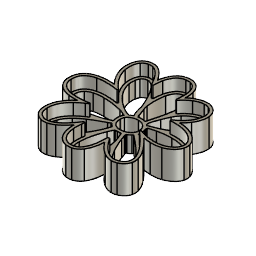
Flower v6 (Autodesk Fusion 360 design; units mm, degrees)
Autodesk Fusion 360 part; units mm, degrees
(part 1 of 2)
sketch "Sketch1" plane through (0, 0, 0) normal (0, 0, 1) x (1, 0, 0)
  spline S0 degree 3 poles (24.398238, -49.491999) (21.853797, -49.043086) (20.145962, -46.595318) (19.808691, -42.913987) knots 0 0 0 0 1 1 1 1
  spline S1 degree 3 poles (19.808691, -42.913987) (19.738303, -42.145705) (19.777142, -40.404034) (19.883263, -39.569933) knots 0 0 0 0 1 1 1 1
  spline S2 degree 3 poles (19.883263, -39.569933) (19.974868, -38.849932) (20.169101, -37.728624) (20.298509, -37.172733) knots 0 0 0 0 1 1 1 1
  spline S3 degree 3 poles (20.298509, -37.172733) (20.350138, -36.950954) (20.383684, -36.760803) (20.373056, -36.750176) knots 0 0 0 0 1 1 1 1
  spline S4 degree 3 poles (20.373056, -36.750176) (20.362429, -36.739548) (20.207496, -36.975057) (20.02876, -37.273529) knots 0 0 0 0 1 1 1 1
  spline S5 degree 3 poles (20.02876, -37.273529) (18.11849, -40.463515) (15.8391, -43.11864) (13.903666, -44.40829) knots 0 0 0 0 1 1 1 1
  spline S6 degree 3 poles (13.903666, -44.40829) (13.13197, -44.9225) (12.4509, -45.23528) (11.669465, -45.434349) knots 0 0 0 0 1 1 1 1
  spline S7 degree 3 poles (11.669465, -45.434349) (11.12034, -45.574233) (10.211189, -45.587693) (9.705467, -45.463417) knots 0 0 0 0 1 1 1 1
  spline S8 degree 3 poles (9.705467, -45.463417) (8.958562, -45.27987) (8.179688, -44.834118) (7.596024, -44.256169) knots 0 0 0 0 1 1 1 1
  spline S9 degree 3 poles (7.596024, -44.256169) (6.902032, -43.568975) (6.551135, -42.561718) (6.474, -41.035376) knots 0 0 0 0 1 1 1 1
  spline S10 degree 3 poles (6.474, -41.035376) (6.338825, -38.360532) (7.582333, -35.682392) (10.063361, -33.304973) knots 0 0 0 0 1 1 1 1
  spline S11 degree 3 poles (10.063361, -33.304973) (10.912309, -32.49148) (11.717344, -31.841911) (12.942719, -30.981678) knots 0 0 0 0 1 1 1 1
  spline S12 degree 3 poles (12.942719, -30.981678) (13.486476, -30.599953) (14.664879, -29.844231) (14.781144, -29.80268) knots 0 0 0 0 1 1 1 1
  spline S13 degree 3 poles (14.781144, -29.80268) (14.813838, -29.790993) (14.829778, -29.770067) (14.816565, -29.756169) knots 0 0 0 0 1 1 1 1
  spline S14 degree 3 poles (14.816565, -29.756169) (14.803352, -29.742275) (14.554706, -29.781213) (14.264021, -29.842704) knots 0 0 0 0 1 1 1 1
  spline S15 degree 3 poles (14.264021, -29.842704) (13.428167, -30.019514) (12.387035, -30.189924) (11.439225, -30.305062) knots 0 0 0 0 1 1 1 1
  spline S16 degree 3 poles (11.439225, -30.305062) (10.694335, -30.39555) (10.318137, -30.411456) (8.906743, -30.412145) knots 0 0 0 0 1 1 1 1
  spline S17 degree 3 poles (8.906743, -30.412145) (7.429716, -30.412867) (7.176998, -30.401447) (6.587244, -30.307359) knots 0 0 0 0 1 1 1 1
  spline S18 degree 3 poles (6.587244, -30.307359) (4.61966, -29.993447) (3.257425, -29.398503) (2.302777, -28.436158) knots 0 0 0 0 1 1 1 1
  spline S19 degree 3 poles (2.302777, -28.436158) (1.404569, -27.53071) (0.964594, -26.480042) (0.898892, -25.083663) knots 0 0 0 0 1 1 1 1
  spline S20 degree 3 poles (0.898892, -25.083663) (0.752423, -21.97074) (2.495588, -19.901678) (5.951833, -19.086041) knots 0 0 0 0 1 1 1 1
  spline S21 degree 3 poles (5.951833, -19.086041) (8.285184, -18.535394) (11.801198, -18.57942) (15.197135, -19.201807) knots 0 0 0 0 1 1 1 1
  spline S22 degree 3 poles (15.197135, -19.201807) (15.472515, -19.252277) (15.706188, -19.285206) (15.71641, -19.274984) knots 0 0 0 0 1 1 1 1
  spline S23 degree 3 poles (15.71641, -19.274984) (15.726633, -19.264761) (15.663483, -19.206281) (15.576077, -19.145026) knots 0 0 0 0 1 1 1 1
  spline S24 degree 3 poles (15.576077, -19.145026) (15.173173, -18.862672) (14.403009, -18.229035) (13.855618, -17.729554) knots 0 0 0 0 1 1 1 1
  spline S25 degree 3 poles (13.855618, -17.729554) (11.319411, -15.415325) (9.535422, -12.521165) (8.985416, -9.828637) knots 0 0 0 0 1 1 1 1
  spline S26 degree 3 poles (8.985416, -9.828637) (8.541535, -7.655641) (8.849932, -5.515577) (9.799961, -4.176243) knots 0 0 0 0 1 1 1 1
  spline S27 degree 3 poles (9.799961, -4.176243) (10.248531, -3.543857) (11.043643, -3.01215) (11.885678, -2.781482) knots 0 0 0 0 1 1 1 1
  spline S28 degree 3 poles (11.885678, -2.781482) (12.362987, -2.650728) (13.37267, -2.662599) (13.879642, -2.804928) knots 0 0 0 0 1 1 1 1
  spline S29 degree 3 poles (13.879642, -2.804928) (16.035873, -3.410271) (18.317612, -5.96279) (20.405058, -10.10473) knots 0 0 0 0 1 1 1 1
  spline S30 degree 3 poles (20.405058, -10.10473) (20.621428, -10.534053) (20.809268, -10.885434) (20.822481, -10.885577) knots 0 0 0 0 1 1 1 1
  spline S31 degree 3 poles (20.822481, -10.885577) (20.835694, -10.88572) (20.839472, -10.577696) (20.830878, -10.201083) knots 0 0 0 0 1 1 1 1
  spline S32 degree 3 poles (20.830878, -10.201083) (20.800341, -8.862913) (20.965717, -7.099114) (21.2307, -5.936803) knots 0 0 0 0 1 1 1 1
  spline S33 degree 3 poles (21.2307, -5.936803) (21.953131, -2.767962) (23.46365, -0.994904) (25.819403, -0.550548) knots 0 0 0 0 1 1 1 1
  spline S34 degree 3 poles (25.819403, -0.550548) (26.276354, -0.464355) (27.303759, -0.478399) (27.762296, -0.577105) knots 0 0 0 0 1 1 1 1
  spline S35 degree 3 poles (27.762296, -0.577105) (29.380756, -0.925504) (30.471677, -2.110585) (30.979854, -4.072385) knots 0 0 0 0 1 1 1 1
  spline S36 degree 3 poles (30.979854, -4.072385) (31.228572, -5.032546) (31.272789, -5.499233) (31.272596, -7.162009) knots 0 0 0 0 1 1 1 1
  spline S37 degree 3 poles (31.272596, -7.162009) (31.272402, -8.704189) (31.219619, -9.467197) (31.030104, -10.666355) knots 0 0 0 0 1 1 1 1
  spline S38 degree 3 poles (31.030104, -10.666355) (30.971872, -11.03482) (30.969098, -11.198786) (31.022394, -11.12191) knots 0 0 0 0 1 1 1 1
  spline S39 degree 3 poles (31.022394, -11.12191) (31.030028, -11.1109) (31.140908, -10.92892) (31.268795, -10.717512) knots 0 0 0 0 1 1 1 1
  spline S40 degree 3 poles (31.268795, -10.717512) (32.09923, -9.344737) (33.682992, -7.788682) (35.140585, -6.913456) knots 0 0 0 0 1 1 1 1
  spline S41 degree 3 poles (35.140585, -6.913456) (36.521936, -6.084012) (37.649445, -5.70804) (38.888276, -5.663775) knots 0 0 0 0 1 1 1 1
  spline S42 degree 3 poles (38.888276, -5.663775) (39.709456, -5.634433) (40.245182, -5.722796) (40.924003, -5.999548) knots 0 0 0 0 1 1 1 1
  spline S43 degree 3 poles (40.924003, -5.999548) (42.412514, -6.606408) (43.266225, -7.780936) (43.456796, -9.48414) knots 0 0 0 0 1 1 1 1
  spline S44 degree 3 poles (43.456796, -9.48414) (43.616225, -10.909023) (42.996088, -13.033743) (41.979428, -14.545917) knots 0 0 0 0 1 1 1 1
  spline S45 degree 3 poles (41.979428, -14.545917) (41.293675, -15.565904) (40.264162, -16.673275) (39.248628, -17.483241) knots 0 0 0 0 1 1 1 1
  spline S46 degree 3 poles (39.248628, -17.483241) (38.697195, -17.92305) (37.559702, -18.70613) (37.002416, -19.02959) knots 0 0 0 0 1 1 1 1
  spline S47 degree 3 poles (37.002416, -19.02959) (36.824039, -19.133123) (36.678096, -19.236237) (36.678096, -19.258731) knots 0 0 0 0 1 1 1 1
  spline S48 degree 3 poles (36.678096, -19.258731) (36.678096, -19.281227) (36.695612, -19.288805) (36.717023, -19.275573) knots 0 0 0 0 1 1 1 1
  spline S49 degree 3 poles (36.717023, -19.275573) (36.738434, -19.262341) (37.173133, -19.217823) (37.68302, -19.176643) knots 0 0 0 0 1 1 1 1
  spline S50 degree 3 poles (37.68302, -19.176643) (42.00013, -18.827983) (45.508277, -19.629245) (47.812293, -21.490171) knots 0 0 0 0 1 1 1 1
  spline S51 degree 3 poles (47.812293, -21.490171) (48.837616, -22.318308) (49.53917, -23.300587) (49.803184, -24.277686) knots 0 0 0 0 1 1 1 1
  spline S52 degree 3 poles (49.803184, -24.277686) (49.942622, -24.793725) (49.943332, -25.611328) (49.80482, -26.123575) knots 0 0 0 0 1 1 1 1
  spline S53 degree 3 poles (49.80482, -26.123575) (49.3646, -27.751308) (47.772047, -29.18037) (45.585744, -29.909516) knots 0 0 0 0 1 1 1 1
  spline S54 degree 3 poles (45.585744, -29.909516) (44.371551, -30.314458) (43.211242, -30.465773) (41.609147, -30.428102) knots 0 0 0 0 1 1 1 1
  spline S55 degree 3 poles (41.609147, -30.428102) (40.042242, -30.391257) (38.585558, -30.162583) (36.798241, -29.672875) knots 0 0 0 0 1 1 1 1
  spline S56 degree 3 poles (36.798241, -29.672875) (36.104288, -29.482739) (34.502045, -28.970831) (34.011496, -28.782527) knots 0 0 0 0 1 1 1 1
  spline S57 degree 3 poles (34.011496, -28.782527) (33.926302, -28.749826) (33.923577, -28.753712) (33.987472, -28.816798) knots 0 0 0 0 1 1 1 1
  spline S58 degree 3 poles (33.987472, -28.816798) (34.027112, -28.855936) (34.286566, -29.080518) (34.56404, -29.315872) knots 0 0 0 0 1 1 1 1
  spline S59 degree 3 poles (34.56404, -29.315872) (37.459824, -31.772092) (40.176255, -34.522567) (41.680793, -36.521819) knots 0 0 0 0 1 1 1 1
  spline S60 degree 3 poles (41.680793, -36.521819) (42.91714, -38.164698) (43.5687, -39.364673) (43.935882, -40.675021) knots 0 0 0 0 1 1 1 1
  spline S61 degree 3 poles (43.935882, -40.675021) (44.082376, -41.197812) (44.118476, -42.215448) (44.008123, -42.711464) knots 0 0 0 0 1 1 1 1
  spline S62 degree 3 poles (44.008123, -42.711464) (43.761857, -43.818382) (42.875081, -44.768754) (41.595179, -45.297459) knots 0 0 0 0 1 1 1 1
  spline S63 degree 3 poles (41.595179, -45.297459) (41.00791, -45.540045) (40.577769, -45.62411) (39.930185, -45.622861) knots 0 0 0 0 1 1 1 1
  spline S64 degree 3 poles (39.930185, -45.622861) (38.88069, -45.620843) (37.959139, -45.323304) (36.774015, -44.603896) knots 0 0 0 0 1 1 1 1
  spline S65 degree 3 poles (36.774015, -44.603896) (34.502488, -43.225002) (32.467553, -40.903967) (30.578279, -37.537086) knots 0 0 0 0 1 1 1 1
  spline S66 degree 3 poles (30.578279, -37.537086) (30.492135, -37.383568) (30.414524, -37.265095) (30.405808, -37.273811) knots 0 0 0 0 1 1 1 1
  spline S67 degree 3 poles (30.405808, -37.273811) (30.397093, -37.282526) (30.409562, -37.559482) (30.433518, -37.889264) knots 0 0 0 0 1 1 1 1
  spline S68 degree 3 poles (30.433518, -37.889264) (30.457475, -38.219047) (30.477736, -39.033089) (30.478545, -39.698245) knots 0 0 0 0 1 1 1 1
  spline S69 degree 3 poles (30.478545, -39.698245) (30.482926, -43.298639) (29.92491, -45.894977) (28.777152, -47.61447) knots 0 0 0 0 1 1 1 1
  spline S70 degree 3 poles (28.777152, -47.61447) (28.158581, -48.54117) (27.313864, -49.174865) (26.365085, -49.423963) knots 0 0 0 0 1 1 1 1
  spline S71 degree 3 poles (26.365085, -49.423963) (25.870005, -49.553947) (24.933082, -49.586358) (24.398238, -49.491999) knots 0 0 0 0 1 1 1 1
  spline S72 degree 3 poles (25.893389, -48.240956) (26.856708, -47.993406) (27.578922, -47.344708) (28.138373, -46.224488) knots 0 0 0 0 1 1 1 1
  spline S73 degree 3 poles (28.138373, -46.224488) (29.483804, -43.53045) (29.645761, -38.006142) (28.50532, -33.708159) knots 0 0 0 0 1 1 1 1
  spline S74 degree 3 poles (28.50532, -33.708159) (28.272808, -32.831887) (28.203024, -32.626149) (27.861593, -31.810289) knots 0 0 0 0 1 1 1 1
  spline S75 degree 3 poles (27.861593, -31.810289) (27.684648, -31.387473) (27.399443, -30.695591) (27.227805, -30.272775) knots 0 0 0 0 1 1 1 1
  spline S76 degree 3 poles (27.227805, -30.272775) (27.056167, -29.849959) (26.901488, -29.489847) (26.884078, -29.47253) knots 0 0 0 0 1 1 1 1
  spline S77 degree 3 poles (26.884078, -29.47253) (26.866667, -29.455214) (26.711883, -29.473809) (26.540113, -29.513859) knots 0 0 0 0 1 1 1 1
  spline S78 degree 3 poles (26.540113, -29.513859) (26.333701, -29.561986) (25.922313, -29.59076) (25.326842, -29.598728) knots 0 0 0 0 1 1 1 1
  line L0 (25.326842, -29.598728) -> (24.425878, -29.610781)
  line L1 (24.425878, -29.610781) -> (24.22792, -29.835671)
  spline S79 degree 3 poles (24.22792, -29.835671) (24.011927, -30.081055) (23.804667, -30.524475) (23.248818, -31.930408) knots 0 0 0 0 1 1 1 1
  spline S80 degree 3 poles (23.248818, -31.930408) (21.722692, -35.790505) (21.010933, -38.900581) (21.011151, -41.708039) knots 0 0 0 0 1 1 1 1
  spline S81 degree 3 poles (21.011151, -41.708039) (21.011248, -43.081883) (21.14664, -44.015287) (21.501171, -45.086507) knots 0 0 0 0 1 1 1 1
  spline S82 degree 3 poles (21.501171, -45.086507) (21.677795, -45.620178) (22.090949, -46.450466) (22.350903, -46.794158) knots 0 0 0 0 1 1 1 1
  spline S83 degree 3 poles (22.350903, -46.794158) (22.951009, -47.587572) (23.718529, -48.09455) (24.573472, -48.262253) knots 0 0 0 0 1 1 1 1
  spline S84 degree 3 poles (24.573472, -48.262253) (24.922627, -48.330746) (25.585621, -48.320048) (25.893389, -48.240956) knots 0 0 0 0 1 1 1 1
  spline S85 degree 3 poles (40.858217, -44.247785) (42.279715, -43.779561) (43.001971, -42.786936) (42.834794, -41.531295) knots 0 0 0 0 1 1 1 1
  spline S86 degree 3 poles (42.834794, -41.531295) (42.633431, -40.018898) (41.504457, -38.100328) (39.382049, -35.663735) knots 0 0 0 0 1 1 1 1
  spline S87 degree 3 poles (39.382049, -35.663735) (38.669928, -34.846195) (36.349413, -32.536002) (35.284727, -31.584633) knots 0 0 0 0 1 1 1 1
  spline S88 degree 3 poles (35.284727, -31.584633) (33.749397, -30.212716) (32.214967, -28.941282) (30.775134, -27.847968) knots 0 0 0 0 1 1 1 1
  line L2 (30.775134, -27.847968) -> (30.181399, -27.397126)
  line L3 (30.181399, -27.397126) -> (29.838211, -27.764149)
  spline S89 degree 3 poles (29.838211, -27.764149) (29.469278, -28.158707) (29.03465, -28.501906) (28.578775, -28.75865) knots 0 0 0 0 1 1 1 1
  spline S90 degree 3 poles (28.578775, -28.75865) (28.422061, -28.846909) (28.286356, -28.924875) (28.27721, -28.931907) knots 0 0 0 0 1 1 1 1
  spline S91 degree 3 poles (28.27721, -28.931907) (28.268063, -28.938939) (28.402431, -29.340808) (28.575805, -29.824947) knots 0 0 0 0 1 1 1 1
  spline S92 degree 3 poles (28.575805, -29.824947) (28.749179, -30.309086) (29.007392, -31.061951) (29.149616, -31.497982) knots 0 0 0 0 1 1 1 1
  spline S93 degree 3 poles (29.149616, -31.497982) (29.589068, -32.845269) (30.956889, -35.77027) (31.924461, -37.431827) knots 0 0 0 0 1 1 1 1
  spline S94 degree 3 poles (31.924461, -37.431827) (33.535773, -40.198841) (35.232289, -42.134083) (37.111751, -43.34905) knots 0 0 0 0 1 1 1 1
  spline S95 degree 3 poles (37.111751, -43.34905) (38.635016, -44.333756) (39.77036, -44.60611) (40.858217, -44.247785) knots 0 0 0 0 1 1 1 1
  spline S96 degree 3 poles (11.005336, -44.276327) (12.706116, -44.048754) (14.648516, -42.571407) (16.719465, -39.930288) knots 0 0 0 0 1 1 1 1
  spline S97 degree 3 poles (16.719465, -39.930288) (18.856844, -37.204452) (20.936605, -33.436523) (21.983766, -30.392893) knots 0 0 0 0 1 1 1 1
  spline S98 degree 3 poles (21.983766, -30.392893) (22.150992, -29.906842) (22.408043, -29.005374) (22.408043, -28.904968) knots 0 0 0 0 1 1 1 1
  spline S99 degree 3 poles (22.408043, -28.904968) (22.408043, -28.885176) (22.287608, -28.78902) (22.140408, -28.691283) knots 0 0 0 0 1 1 1 1
  spline S100 degree 3 poles (22.140408, -28.691283) (21.993209, -28.593549) (21.695916, -28.334201) (21.479758, -28.114959) knots 0 0 0 0 1 1 1 1
  line L4 (21.479758, -28.114959) -> (21.086741, -27.716331)
  line L5 (21.086741, -27.716331) -> (20.846504, -27.859244)
  spline S101 degree 3 poles (20.846504, -27.859244) (20.714374, -27.937846) (20.292759, -28.164898) (19.909582, -28.363802) knots 0 0 0 0 1 1 1 1
  spline S102 degree 3 poles (19.909582, -28.363802) (17.754742, -29.482369) (15.357081, -30.859413) (14.095855, -31.70279) knots 0 0 0 0 1 1 1 1
  spline S103 degree 3 poles (14.095855, -31.70279) (12.638315, -32.677443) (11.799362, -33.354871) (10.753846, -34.401361) knots 0 0 0 0 1 1 1 1
  spline S104 degree 3 poles (10.753846, -34.401361) (9.338842, -35.817684) (8.596538, -36.929435) (8.095304, -38.383066) knots 0 0 0 0 1 1 1 1
  spline S105 degree 3 poles (8.095304, -38.383066) (7.64097, -39.700685) (7.580163, -41.336302) (7.942137, -42.503075) knots 0 0 0 0 1 1 1 1
  spline S106 degree 3 poles (7.942137, -42.503075) (8.124894, -43.092168) (8.614245, -43.621961) (9.291121, -43.963548) knots 0 0 0 0 1 1 1 1
  spline S107 degree 3 poles (9.291121, -43.963548) (9.729941, -44.184998) (10.00671, -44.262128) (10.57291, -44.320759) knots 0 0 0 0 1 1 1 1
  spline S108 degree 3 poles (10.57291, -44.320759) (10.604031, -44.323982) (10.798622, -44.303987) (11.005336, -44.276327) knots 0 0 0 0 1 1 1 1
  spline S109 degree 3 poles (9.86769, -29.190267) (11.999504, -29.071706) (14.228262, -28.682383) (16.330056, -28.061413) knots 0 0 0 0 1 1 1 1
  spline S110 degree 3 poles (16.330056, -28.061413) (17.685108, -27.661063) (18.407858, -27.389856) (19.490909, -26.875315) knots 0 0 0 0 1 1 1 1
  spline S111 degree 3 poles (19.490909, -26.875315) (20.05102, -26.609216) (20.231482, -26.543822) (20.34375, -26.566274) knots 0 0 0 0 1 1 1 1
  spline S112 degree 3 poles (20.34375, -26.566274) (20.511378, -26.599799) (20.510381, -26.60631) (20.394298, -26.236136) knots 0 0 0 0 1 1 1 1
  spline S113 degree 3 poles (20.394298, -26.236136) (20.208637, -25.644081) (20.136723, -25.011267) (20.163424, -24.204533) knots 0 0 0 0 1 1 1 1
  spline S114 degree 3 poles (20.163424, -24.204533) (20.191288, -23.362655) (20.251637, -23.079623) (20.524075, -22.513134) knots 0 0 0 0 1 1 1 1
  spline S115 degree 3 poles (20.524075, -22.513134) (20.619391, -22.314939) (20.704187, -22.141122) (20.712509, -22.126876) knots 0 0 0 0 1 1 1 1
  spline S116 degree 3 poles (20.712509, -22.126876) (20.720832, -22.112629) (20.624658, -22.07382) (20.498789, -22.040629) knots 0 0 0 0 1 1 1 1
  spline S117 degree 3 poles (20.498789, -22.040629) (20.37292, -22.007438) (20.010481, -21.853011) (19.693369, -21.697453) knots 0 0 0 0 1 1 1 1
  spline S118 degree 3 poles (19.693369, -21.697453) (19.031376, -21.37272) (18.940258, -21.339975) (17.963665, -21.075839) knots 0 0 0 0 1 1 1 1
  spline S119 degree 3 poles (17.963665, -21.075839) (15.215646, -20.332598) (12.511082, -19.953422) (9.915737, -19.947536) knots 0 0 0 0 1 1 1 1
  spline S120 degree 3 poles (9.915737, -19.947536) (8.066739, -19.943341) (6.90521, -20.076177) (5.769446, -20.421715) knots 0 0 0 0 1 1 1 1
  spline S121 degree 3 poles (5.769446, -20.421715) (4.597844, -20.778155) (3.959645, -21.127141) (3.306742, -21.768398) knots 0 0 0 0 1 1 1 1
  spline S122 degree 3 poles (3.306742, -21.768398) (2.424956, -22.634452) (2.095276, -23.542207) (2.14632, -24.963545) knots 0 0 0 0 1 1 1 1
  spline S123 degree 3 poles (2.14632, -24.963545) (2.175414, -25.773698) (2.241396, -26.057452) (2.544106, -26.67421) knots 0 0 0 0 1 1 1 1
  spline S124 degree 3 poles (2.544106, -26.67421) (3.271215, -28.155669) (5.031283, -28.989333) (7.849702, -29.187235) knots 0 0 0 0 1 1 1 1
  spline S125 degree 3 poles (7.849702, -29.187235) (8.663341, -29.244367) (8.888833, -29.244704) (9.86769, -29.190267) knots 0 0 0 0 1 1 1 1
  spline S126 degree 3 poles (43.332654, -29.137953) (45.833001, -28.886581) (48.03311, -27.538142) (48.575731, -25.924491) knots 0 0 0 0 1 1 1 1
  spline S127 degree 3 poles (48.575731, -25.924491) (48.63969, -25.734282) (48.663866, -25.525594) (48.66199, -25.179758) knots 0 0 0 0 1 1 1 1
  spline S128 degree 3 poles (48.66199, -25.179758) (48.659731, -24.761074) (48.640646, -24.652073) (48.513666, -24.332161) knots 0 0 0 0 1 1 1 1
  spline S129 degree 3 poles (48.513666, -24.332161) (48.302063, -23.799048) (47.985644, -23.355484) (47.45205, -22.843943) knots 0 0 0 0 1 1 1 1
  spline S130 degree 3 poles (47.45205, -22.843943) (46.86571, -22.281845) (46.265738, -21.868736) (45.50635, -21.504241) knots 0 0 0 0 1 1 1 1
  spline S131 degree 3 poles (45.50635, -21.504241) (43.811723, -20.690849) (42.068315, -20.351389) (39.58496, -20.351283) knots 0 0 0 0 1 1 1 1
  spline S132 degree 3 poles (39.58496, -20.351283) (37.563224, -20.351186) (35.890814, -20.547427) (33.675071, -21.044717) knots 0 0 0 0 1 1 1 1
  spline S133 degree 3 poles (33.675071, -21.044717) (32.283276, -21.357085) (30.762301, -21.829765) (30.583775, -22.005414) knots 0 0 0 0 1 1 1 1
  spline S134 degree 3 poles (30.583775, -22.005414) (30.529994, -22.05833) (30.53212, -22.093371) (30.596693, -22.218237) knots 0 0 0 0 1 1 1 1
  spline S135 degree 3 poles (30.596693, -22.218237) (30.641341, -22.304578) (30.670547, -22.465069) (30.665834, -22.598196) knots 0 0 0 0 1 1 1 1
  spline S136 degree 3 poles (30.665834, -22.598196) (30.661347, -22.72496) (30.681981, -22.874087) (30.711685, -22.929592) knots 0 0 0 0 1 1 1 1
  spline S137 degree 3 poles (30.711685, -22.929592) (30.741389, -22.985094) (30.821132, -23.243824) (30.888889, -23.504541) knots 0 0 0 0 1 1 1 1
  spline S138 degree 3 poles (30.888889, -23.504541) (31.059524, -24.161122) (31.093911, -24.851664) (30.987623, -25.487306) knots 0 0 0 0 1 1 1 1
  spline S139 degree 3 poles (30.987623, -25.487306) (30.942203, -25.758936) (30.912106, -25.988237) (30.920742, -25.996867) knots 0 0 0 0 1 1 1 1
  spline S140 degree 3 poles (30.920742, -25.996867) (30.929379, -26.005495) (31.358057, -26.229394) (31.873366, -26.494417) knots 0 0 0 0 1 1 1 1
  spline S141 degree 3 poles (31.873366, -26.494417) (34.111623, -27.645556) (37.397061, -28.703659) (39.801175, -29.047629) knots 0 0 0 0 1 1 1 1
  spline S142 degree 3 poles (39.801175, -29.047629) (41.093914, -29.23259) (42.128198, -29.259045) (43.332654, -29.137953) knots 0 0 0 0 1 1 1 1
  spline S143 degree 3 poles (26.591706, -28.217443) (28.144132, -27.809112) (29.245549, -26.902497) (29.669204, -25.684255) knots 0 0 0 0 1 1 1 1
  spline S144 degree 3 poles (29.669204, -25.684255) (29.811671, -25.274583) (29.826821, -24.33512) (29.698515, -23.866764) knots 0 0 0 0 1 1 1 1
  spline S145 degree 3 poles (29.698515, -23.866764) (29.469369, -23.03032) (29.247409, -22.592355) (28.85237, -22.197175) knots 0 0 0 0 1 1 1 1
  spline S146 degree 3 poles (28.85237, -22.197175) (27.955357, -21.299841) (26.950574, -20.869384) (25.750353, -20.868248) knots 0 0 0 0 1 1 1 1
  spline S147 degree 3 poles (25.750353, -20.868248) (23.94356, -20.866537) (22.347837, -21.673224) (21.723986, -22.9037) knots 0 0 0 0 1 1 1 1
  spline S148 degree 3 poles (21.723986, -22.9037) (21.471631, -23.401441) (21.399039, -23.732455) (21.399116, -24.385059) knots 0 0 0 0 1 1 1 1
  spline S149 degree 3 poles (21.399116, -24.385059) (21.399357, -26.530244) (22.466498, -27.923444) (24.40201, -28.305518) knots 0 0 0 0 1 1 1 1
  spline S150 degree 3 poles (24.40201, -28.305518) (24.938571, -28.411436) (26.019466, -28.367961) (26.591706, -28.217443) knots 0 0 0 0 1 1 1 1
  spline S151 degree 3 poles (30.655206, -20.5982) (33.956991, -19.389184) (36.517221, -18.055607) (38.383779, -16.572527) knots 0 0 0 0 1 1 1 1
  spline S152 degree 3 poles (38.383779, -16.572527) (40.429873, -14.946796) (41.641989, -13.166128) (42.110688, -11.097479) knots 0 0 0 0 1 1 1 1
  spline S153 degree 3 poles (42.110688, -11.097479) (42.194568, -10.72726) (42.218598, -10.471865) (42.218771, -9.948755) knots 0 0 0 0 1 1 1 1
  spline S154 degree 3 poles (42.218771, -9.948755) (42.218964, -9.35041) (42.204926, -9.233209) (42.091661, -8.887946) knots 0 0 0 0 1 1 1 1
  spline S155 degree 3 poles (42.091661, -8.887946) (41.79982, -7.998312) (41.17612, -7.39316) (40.209114, -7.061391) knots 0 0 0 0 1 1 1 1
  spline S156 degree 3 poles (40.209114, -7.061391) (39.696089, -6.885378) (38.825126, -6.845508) (38.214306, -6.970076) knots 0 0 0 0 1 1 1 1
  spline S157 degree 3 poles (38.214306, -6.970076) (36.572591, -7.304878) (34.717053, -8.472871) (33.291384, -10.068873) knots 0 0 0 0 1 1 1 1
  spline S158 degree 3 poles (33.291384, -10.068873) (32.670957, -10.763426) (32.104538, -11.643131) (31.605352, -12.687453) knots 0 0 0 0 1 1 1 1
  spline S159 degree 3 poles (31.605352, -12.687453) (31.202006, -13.531272) (31.008397, -14.002414) (30.302233, -15.858576) knots 0 0 0 0 1 1 1 1
  spline S160 degree 3 poles (30.302233, -15.858576) (29.172382, -18.828409) (28.914262, -19.794926) (29.057562, -20.519167) knots 0 0 0 0 1 1 1 1
  spline S161 degree 3 poles (29.057562, -20.519167) (29.085668, -20.66122) (29.15393, -20.763894) (29.319224, -20.912747) knots 0 0 0 0 1 1 1 1
  spline S162 degree 3 poles (29.319224, -20.912747) (29.538915, -21.110584) (29.544555, -21.112558) (29.639057, -21.024597) knots 0 0 0 0 1 1 1 1
  spline S163 degree 3 poles (29.639057, -21.024597) (29.691967, -20.97535) (30.149231, -20.783471) (30.655201, -20.5982) knots 0 0 0 0 1 1 1 1
  spline S164 degree 3 poles (21.920657, -20.791021) (22.126118, -20.630778) (22.605845, -20.349544) (22.82846, -20.258832) knots 0 0 0 0 1 1 1 1
  spline S165 degree 3 poles (22.82846, -20.258832) (22.914343, -20.223835) (22.984614, -20.183399) (22.984614, -20.168972) knots 0 0 0 0 1 1 1 1
  spline S166 degree 3 poles (22.984614, -20.168972) (22.984614, -20.154545) (22.868126, -19.913929) (22.725752, -19.634268) knots 0 0 0 0 1 1 1 1
  spline S167 degree 3 poles (22.725752, -19.634268) (22.304419, -18.80666) (21.962693, -17.821308) (21.610188, -16.417587) knots 0 0 0 0 1 1 1 1
  spline S168 degree 3 poles (21.610188, -16.417587) (21.49406, -15.955162) (21.399049, -15.536827) (21.399049, -15.487954) knots 0 0 0 0 1 1 1 1
  spline S169 degree 3 poles (21.399049, -15.487954) (21.399049, -15.188889) (20.490535, -13.054965) (19.572604, -11.197985) knots 0 0 0 0 1 1 1 1
  spline S170 degree 3 poles (19.572604, -11.197985) (17.226619, -6.452048) (14.886759, -3.920235) (12.846624, -3.920235) knots 0 0 0 0 1 1 1 1
  spline S171 degree 3 poles (12.846624, -3.920235) (11.939436, -3.920235) (11.101435, -4.383869) (10.643793, -5.138975) knots 0 0 0 0 1 1 1 1
  spline S172 degree 3 poles (10.643793, -5.138975) (10.443402, -5.469619) (10.239039, -6.078373) (10.125946, -6.681536) knots 0 0 0 0 1 1 1 1
  spline S173 degree 3 poles (10.125946, -6.681536) (10.005281, -7.325079) (10.00555, -8.696807) (10.126465, -9.32414) knots 0 0 0 0 1 1 1 1
  spline S174 degree 3 poles (10.126465, -9.32414) (10.490692, -11.213843) (11.35488, -12.995203) (12.771902, -14.777209) knots 0 0 0 0 1 1 1 1
  spline S175 degree 3 poles (12.771902, -14.777209) (13.302785, -15.444832) (14.606985, -16.776276) (15.273017, -17.330568) knots 0 0 0 0 1 1 1 1
  spline S176 degree 3 poles (15.273017, -17.330568) (16.713493, -18.529377) (19.047161, -20.032692) (20.066455, -20.418432) knots 0 0 0 0 1 1 1 1
  spline S177 degree 3 poles (20.066455, -20.418432) (20.231224, -20.480787) (20.549816, -20.609314) (20.774436, -20.704051) knots 0 0 0 0 1 1 1 1
  spline S178 degree 3 poles (20.774436, -20.704051) (21.089287, -20.836843) (21.222917, -20.869949) (21.357799, -20.848579) knots 0 0 0 0 1 1 1 1
  spline S179 degree 3 poles (21.357799, -20.848579) (21.454027, -20.833334) (21.572945, -20.844211) (21.622059, -20.872754) knots 0 0 0 0 1 1 1 1
  spline S180 degree 3 poles (21.622059, -20.872754) (21.740008, -20.941295) (21.721474, -20.946369) (21.920657, -20.791021) knots 0 0 0 0 1 1 1 1
  spline S181 degree 3 poles (27.658011, -19.803937) (27.645958, -19.740885) (27.798939, -19.130083) (27.997973, -18.4466) knots 0 0 0 0 1 1 1 1
  spline S182 degree 3 poles (27.997973, -18.4466) (29.529616, -13.186856) (30.181548, -9.34461) (30.047201, -6.369229) knots 0 0 0 0 1 1 1 1
  spline S183 degree 3 poles (30.047201, -6.369229) (30.008787, -5.518475) (30.001195, -5.448311) (29.873024, -4.759643) knots 0 0 0 0 1 1 1 1
  spline S184 degree 3 poles (29.873024, -4.759643) (29.570027, -3.13163) (28.823901, -2.149445) (27.641773, -1.822471) knots 0 0 0 0 1 1 1 1
  spline S185 degree 3 poles (27.641773, -1.822471) (27.171406, -1.692367) (26.203629, -1.704005) (25.702006, -1.845797) knots 0 0 0 0 1 1 1 1
  spline S186 degree 3 poles (25.702006, -1.845797) (24.127691, -2.290803) (23.064336, -3.652227) (22.505903, -5.937794) knots 0 0 0 0 1 1 1 1
  spline S187 degree 3 poles (22.505903, -5.937794) (21.987577, -8.059213) (21.925904, -10.946323) (22.339221, -13.740611) knots 0 0 0 0 1 1 1 1
  spline S188 degree 3 poles (22.339221, -13.740611) (22.484785, -14.724719) (22.468031, -14.661766) (22.836169, -15.607863) knots 0 0 0 0 1 1 1 1
  spline S189 degree 3 poles (22.836169, -15.607863) (23.19607, -16.532792) (23.711209, -17.972242) (24.017763, -18.909582) knots 0 0 0 0 1 1 1 1
  spline S190 degree 3 poles (24.017763, -18.909582) (24.143081, -19.292759) (24.273962, -19.636492) (24.30861, -19.673434) knots 0 0 0 0 1 1 1 1
  spline S191 degree 3 poles (24.30861, -19.673434) (24.361523, -19.729847) (24.430723, -19.731064) (24.740837, -19.681037) knots 0 0 0 0 1 1 1 1
  spline S192 degree 3 poles (24.740837, -19.681037) (25.528811, -19.553923) (26.915972, -19.64906) (27.461185, -19.867609) knots 0 0 0 0 1 1 1 1
  spline S193 degree 3 poles (27.461185, -19.867609) (27.641588, -19.939923) (27.681539, -19.927001) (27.658011, -19.803937) knots 0 0 0 0 1 1 1 1
  spline S194 degree 3 poles (14.203993, -1.649594) (15.876078, -2.119017) (17.363844, -3.374033) (18.770183, -5.177884) (19.141135, -5.65369) (19.506115, -6.170373) (19.865458, -6.727006) knots 0.00000016 0.00000016 0.00000016 0.00000016 0.59946487 0.59946487 0.59946487 0.7575867 0.7575867 0.7575867 0.7575867
  spline S195 degree 3 poles (19.865458, -6.727006) (19.921486, -6.352401) (19.98592, -5.998167) (20.060719, -5.670071) knots 0.75017991 0.75017991 0.75017991 0.75017991 1 1 1 1
  spline S196 degree 3 poles (20.060719, -5.670071) (20.539039, -3.57199) (21.368047, -1.896529) (22.668932, -0.765695) (23.49334, -0.049053) (24.497154, 0.421203) (25.596974, 0.628658) knots 0 0 0 0 0.61209687 0.61209687 0.61209687 1 1 1 1
  spline S197 degree 3 poles (25.596974, 0.628658) (25.956294, 0.696435) (26.298777, 0.706584) (26.675131, 0.706342) (27.071573, 0.706087) (27.463404, 0.687562) (27.827195, 0.63056) (27.889104, 0.620859) (27.950904, 0.609782) (28.014829, 0.596022) knots 0 0 0 0 0.44790095 0.44790095 0.44790095 0.91970835 0.91970835 0.91970835 1 1 1 1
  spline S198 degree 3 poles (28.01483, 0.596021) (29.367827, 0.304768) (30.525995, -0.5171) (31.269202, -1.691236) (31.656083, -2.30244) (31.941823, -3.000576) (32.141514, -3.771474) knots 0 0 0 0 0.65765407 0.65765407 0.65765407 1 1 1 1
  spline S199 degree 3 poles (32.141514, -3.771474) (32.348926, -4.572177) (32.443264, -5.202689) (32.464816, -6.218515) (32.470667, -6.494335) (32.472638, -6.802529) (32.472596, -7.162149) knots 0.00000048 0.00000048 0.00000048 0.00000048 0.78645882 0.78645882 0.78645882 1 1 1 1
  spline S200 degree 3 poles (32.472596, -7.16216) (32.472584, -7.259473) (32.472367, -7.353735) (32.471919, -7.445993) knots 0 0 0 0 0.06200234 0.06200234 0.06200234 0.06200234
  spline S201 degree 3 poles (32.471919, -7.445993) (32.917086, -7.035403) (33.387025, -6.651534) (33.865633, -6.314097) (34.082904, -6.160913) (34.302176, -6.017175) (34.522842, -5.884673) knots 0.57599496 0.57599496 0.57599496 0.57599496 0.86761491 0.86761491 0.86761491 1 1 1 1
  spline S202 degree 3 poles (34.522843, -5.884673) (36.014058, -4.989261) (37.390234, -4.516536) (38.845426, -4.46454) knots 0 0 0 0 1 1 1 1
  spline S203 degree 3 poles (38.845426, -4.46454) (39.771138, -4.431463) (40.576517, -4.561982) (41.377034, -4.88835) knots 0.00000004 0.00000004 0.00000004 0.00000004 1 1 1 1
  spline S204 degree 3 poles (41.377034, -4.88835) (42.666561, -5.414084) (43.684375, -6.380736) (44.212711, -7.628784) (44.438742, -8.162718) (44.58109, -8.740601) (44.649354, -9.350705) knots 0 0 0 0 0.70037073 0.70037073 0.70037073 1 1 1 1
  spline S205 degree 3 poles (44.649354, -9.350705) (44.784456, -10.558164) (44.517866, -11.869945) (44.034754, -13.142071) (43.758612, -13.869203) (43.40481, -14.576573) (42.975284, -15.215447) knots 0.00000002 0.00000002 0.00000002 0.00000002 0.6362988 0.6362988 0.6362988 1 1 1 1
  spline S206 degree 3 poles (42.975284, -15.215447) (42.340878, -16.15906) (41.493587, -17.110225) (40.590265, -17.91902) knots 0.00000005 0.00000005 0.00000005 0.00000005 0.82214228 0.82214228 0.82214228 0.82214228
  spline S207 degree 3 poles (40.590265, -17.91902) (43.45697, -18.048348) (45.945261, -18.743579) (47.896164, -20.061461) (48.127628, -20.217821) (48.351181, -20.382895) (48.566295, -20.556639) knots 0.23064134 0.23064134 0.23064134 0.23064134 0.91840095 0.91840095 0.91840095 1 1 1 1
  spline S208 degree 3 poles (48.566295, -20.556639) (49.744301, -21.508098) (50.610818, -22.666298) (50.96164, -23.964669) knots 0.00000047 0.00000047 0.00000047 0.00000047 1 1 1 1
  spline S209 degree 3 poles (50.96164, -23.964669) (51.124068, -24.565794) (51.140844, -25.172463) (51.080545, -25.773981) (51.058271, -25.996182) (51.02331, -26.214573) (50.963219, -26.436805) (50.963216, -26.436815) (50.963214, -26.436824) (50.963211, -26.436833) knots 0.0000028 0.0000028 0.0000028 0.0000028 0.73024687 0.73024687 0.73024687 1 1 1 1.00001792 1.00001792 1.00001792 1.00001792
  spline S210 degree 3 poles (50.963211, -26.436833) (50.963209, -26.436842) (50.963206, -26.436851) (50.963204, -26.436861) (50.519992, -28.075651) (49.271077, -29.40819) (47.641897, -30.314192) (47.122818, -30.602856) (46.561441, -30.849092) (45.965395, -31.047877) knots -0.00000564 -0.00000564 -0.00000564 -0.00000564 0 0 0 0.75837207 0.75837207 0.75837207 1 1 1 1
  spline S211 degree 3 poles (45.965395, -31.047877) (44.618653, -31.497025) (43.272142, -31.667537) (41.580938, -31.62777) knots 0.00000011 0.00000011 0.00000011 0.00000011 1 1 1 1
  spline S212 degree 3 poles (41.580937, -31.62777) (40.567212, -31.603933) (39.584175, -31.503217) (38.553365, -31.312101) knots 0 0 0 0 0.60844734 0.60844734 0.60844734 0.60844734
  spline S213 degree 3 poles (38.553365, -31.312101) (40.206304, -32.912548) (41.642718, -34.475561) (42.639617, -35.800255) knots 0.37843695 0.37843695 0.37843695 0.37843695 1 1 1 1
  spline S214 degree 3 poles (42.639618, -35.800255) (43.922977, -37.505603) (44.676032, -38.869017) (45.091374, -40.351233) knots 0 0 0 0 1 1 1 1
  spline S215 degree 3 poles (45.091374, -40.351235) (45.223275, -40.821945) (45.261103, -41.294339) (45.270967, -41.782869) (45.279189, -42.190068) (45.269477, -42.567564) (45.179484, -42.972066) knots 0 0 0 0 0.54539945 0.54539945 0.54539945 1 1 1 1
  spline S216 degree 3 poles (45.179484, -42.972067) (44.856208, -44.42513) (43.780089, -45.591165) (42.372532, -46.264469) (42.268086, -46.314431) (42.161651, -46.361811) (42.053328, -46.406558) knots 0 0 0 0 0.93092246 0.93092246 0.93092246 1 1 1 1
  spline S217 degree 3 poles (42.05332, -46.406561) (41.365365, -46.690737) (40.680329, -46.82431) (39.92787, -46.822859) knots 0 0 0 0 1 1 1 1
  spline S218 degree 3 poles (39.92787, -46.822859) (38.815354, -46.820718) (37.742242, -46.513782) (36.63982, -45.911774) (36.478865, -45.82388) (36.316378, -45.729885) (36.151325, -45.629692) knots 0.0000021 0.0000021 0.0000021 0.0000021 0.87259897 0.87259897 0.87259897 1 1 1 1
  spline S219 degree 3 poles (36.151323, -45.629691) (34.509624, -44.633123) (33.018363, -43.215897) (31.637272, -41.383046) knots 0 0 0 0 0.65396261 0.65396261 0.65396261 0.65396261
  spline S220 degree 3 poles (31.637272, -41.383046) (31.494286, -44.103071) (30.98906, -46.27158) (29.984476, -47.949714) (29.917006, -48.062423) (29.847265, -48.172766) (29.77523, -48.280684) knots 0.15697726 0.15697726 0.15697726 0.15697726 0.94694366 0.94694366 0.94694366 1 1 1 1
  spline S221 degree 3 poles (29.775229, -48.280685) (29.016834, -49.416859) (27.932868, -50.253016) (26.669813, -50.584627) knots 0 0 0 0 1 1 1 1
  spline S222 degree 3 poles (26.669813, -50.584627) (26.214933, -50.704056) (25.755317, -50.73828) (25.276254, -50.745394) (24.905035, -50.750906) (24.546559, -50.736698) (24.189751, -50.673749) knots 0.0000016 0.0000016 0.0000016 0.0000016 0.56341737 0.56341737 0.56341737 1 1 1 1
  spline S223 degree 3 poles (24.189744, -50.673748) (22.560867, -50.386367) (21.174019, -49.407066) (20.231405, -48.014131) (19.328589, -46.680005) (18.792964, -44.980199) (18.613695, -43.023469) knots 0 0 0 0 0.51078259 0.51078259 0.51078259 1 1 1 1
  spline S224 degree 3 poles (18.613695, -43.023469) (18.574975, -42.600839) (18.567986, -42.065666) (18.575476, -41.49903) knots 0.00000013 0.00000013 0.00000013 0.00000013 0.43466848 0.43466848 0.43466848 0.43466848
  spline S225 degree 3 poles (18.575476, -41.49903) (17.596183, -42.734487) (16.591639, -43.800646) (15.598078, -44.631736) (15.254546, -44.919092) (14.911886, -45.178477) (14.569077, -45.406903) knots 0.39518925 0.39518925 0.39518925 0.39518925 0.84460942 0.84460942 0.84460942 1 1 1 1
  spline S226 degree 3 poles (14.569077, -45.406903) (13.713118, -45.977261) (12.87689, -46.365086) (11.965701, -46.597209) knots 0.00000026 0.00000026 0.00000026 0.00000026 1 1 1 1
  spline S227 degree 3 poles (11.965692, -46.597212) (11.387538, -46.74449) (10.786586, -46.771883) (10.200068, -46.73762) (9.93614, -46.722202) (9.682541, -46.693485) (9.419098, -46.628746) knots 0 0 0 0 0.68965977 0.68965977 0.68965977 1 1 1 1
  spline S228 degree 3 poles (9.419095, -46.628745) (8.422699, -46.383888) (7.495413, -45.845312) (6.751681, -45.108861) knots 0 0 0 0 1 1 1 1
  spline S229 degree 3 poles (6.751681, -45.108861) (6.024456, -44.38876) (5.591289, -43.408642) (5.399734, -42.278186) (5.336609, -41.90565) (5.29661, -41.513089) (5.275529, -41.095942) knots 0.00000071 0.00000071 0.00000071 0.00000071 0.7521372 0.7521372 0.7521372 1 1 1 1
  spline S230 degree 3 poles (5.275529, -41.095942) (5.134749, -38.310175) (6.307323, -35.5678) (8.492197, -33.193771) (8.727402, -32.938203) (8.974453, -32.686409) (9.233117, -32.438547) knots 0 0 0 0 0.90281087 0.90281087 0.90281087 1 1 1 1
  spline S231 degree 3 poles (9.233118, -32.438546) (9.537673, -32.14671) (9.84093, -31.871196) (10.15681, -31.601569) knots 0 0 0 0 0.34136527 0.34136527 0.34136527 0.34136527
  spline S232 degree 3 poles (10.15681, -31.601569) (9.933711, -31.607004) (9.687499, -31.609728) (9.387832, -31.611081) (9.240949, -31.611744) (9.081721, -31.61206) (8.907329, -31.612145) knots 0.62671458 0.62671458 0.62671458 0.62671458 0.87721557 0.87721557 0.87721557 1 1 1 1
  spline S233 degree 3 poles (8.907329, -31.612145) (7.809609, -31.612681) (7.343172, -31.608321) (6.878045, -31.558344) (6.714675, -31.54079) (6.5613, -31.518395) (6.398188, -31.492372) knots 0.00000004 0.00000004 0.00000004 0.00000004 0.7400635 0.7400635 0.7400635 1 1 1 1
  spline S234 degree 3 poles (6.398185, -31.492372) (4.455271, -31.182396) (2.911566, -30.58943) (1.750221, -29.563762) (1.647099, -29.472688) (1.547282, -29.378484) (1.450848, -29.281272) knots 0 0 0 0 0.91844647 0.91844647 0.91844647 1 1 1 1
  spline S235 degree 3 poles (1.450848, -29.281272) (0.525731, -28.348698) (-0.052564, -27.173435) (-0.235266, -25.849544) (-0.267255, -25.617741) (-0.288429, -25.381356) (-0.299782, -25.140063) knots 0.00000029 0.00000029 0.00000029 0.00000029 0.85099689 0.85099689 0.85099689 1 1 1 1
  spline S236 degree 3 poles (-0.299782, -25.140063) (-0.382779, -23.376118) (0.083649, -21.756259) (1.107088, -20.50976) (2.16329, -19.223358) (3.741213, -18.374762) (5.676216, -17.918121) knots 0.00000001 0.00000001 0.00000001 0.00000001 0.49212315 0.49212315 0.49212315 1 1 1 1
  spline S237 degree 3 poles (5.676216, -17.918121) (7.441319, -17.501575) (9.651698, -17.410094) (11.995177, -17.583099) knots 0.00000003 0.00000003 0.00000003 0.00000003 0.67640459 0.67640459 0.67640459 0.67640459
  spline S238 degree 3 poles (11.995177, -17.583099) (9.857007, -15.321979) (8.344019, -12.684563) (7.809695, -10.068803) knots 0.135529 0.135529 0.135529 0.135529 1 1 1 1
  spline S239 degree 3 poles (7.809695, -10.068803) (7.383214, -7.980989) (7.544378, -5.907835) (8.360502, -4.257492) (8.494712, -3.986098) (8.647751, -3.726486) (8.821191, -3.481973) knots 0.00000001 0.00000001 0.00000001 0.00000001 0.85877638 0.85877638 0.85877638 1 1 1 1
  spline S240 degree 3 poles (8.821191, -3.481973) (9.438052, -2.612334) (10.355489, -2.00156) (11.39012, -1.676601) (11.449191, -1.658047) (11.508701, -1.640539) (11.56863, -1.624122) knots 0 0 0 0 0.9459899 0.9459899 0.9459899 1 1 1 1
  spline S241 degree 3 poles (11.568631, -1.624122) (11.971813, -1.513674) (12.335824, -1.494343) (12.731334, -1.490683) (13.179919, -1.486531) (13.622212, -1.513049) (14.057883, -1.612546) (14.106084, -1.623554) (14.154601, -1.635728) (14.203993, -1.649594) knots 0 0 0 0 0.44254044 0.44254044 0.44254044 0.94446886 0.94446886 0.94446886 1 1 1 1
  line L6 (32.472573, -7.085931) -> (32.471919, -7.445993)
  spline S242 degree 3 poles (32.774528, -45.054803) (32.597745, -45.852669) (32.369356, -46.608949) (32.077654, -47.322455) (31.810229, -47.976577) (31.488921, -48.595303) (31.105999, -49.16897) knots 0.51113009 0.51113009 0.51113009 0.51113009 0.76617847 0.76617847 0.76617847 1 1 1 1
  spline S243 degree 3 poles (31.105998, -49.168972) (30.161172, -50.584444) (28.758206, -51.690552) (27.076118, -52.132179) knots 0 0 0 0 1 1 1 1
  spline S244 degree 3 poles (27.076118, -52.132179) (26.570504, -52.264927) (26.177275, -52.301703) (25.75781, -52.327692) (25.262853, -52.358359) (24.781509, -52.359093) (24.249906, -52.298187) (24.141641, -52.285783) (24.030309, -52.270329) (23.911771, -52.249416) knots 0.00000246 0.00000246 0.00000246 0.00000246 0.41317546 0.41317546 0.41317546 0.90070894 0.90070894 0.90070894 0.99999884 0.99999884 0.99999884 0.99999884
  spline S245 degree 3 poles (23.911771, -52.249416) (23.911765, -52.249415) (23.911758, -52.249414) (23.911751, -52.249413) (22.213686, -51.949825) (20.678346, -51.034136) (19.573633, -49.776284) (18.465941, -48.515042) (17.751636, -46.954394) (17.346823, -45.219075) knots -0.00000266 -0.00000266 -0.00000266 -0.00000266 0 0 0 0.41944391 0.41944391 0.41944391 0.84001856 0.84001856 0.84001856 0.84001856
  spline S246 degree 3 poles (17.346823, -45.219075) (16.732734, -45.793276) (16.108772, -46.303616) (15.456293, -46.738386) knots 0.7458211 0.7458211 0.7458211 0.7458211 1 1 1 1
  spline S247 degree 3 poles (15.456293, -46.738386) (14.487982, -47.383608) (13.444876, -47.871493) (12.360684, -48.147689) knots 0.00000054 0.00000054 0.00000054 0.00000054 1 1 1 1
  spline S248 degree 3 poles (12.360681, -48.14769) (12.360675, -48.147692) (12.360668, -48.147693) (12.360662, -48.147695) (11.740561, -48.305659) (11.228823, -48.341283) (10.691453, -48.347924) (10.228916, -48.35364) (9.784254, -48.335181) (9.253446, -48.230312) (9.183769, -48.216546) (9.112059, -48.200897) (9.037272, -48.182519) knots -0.00001192 -0.00001192 -0.00001192 -0.00001192 0 0 0 0.50665603 0.50665603 0.50665603 0.94275511 0.94275511 0.94275511 1 1 1 1
  spline S249 degree 3 poles (9.037266, -48.182517) (7.830329, -47.88592) (6.796578, -47.305624) (5.894737, -46.498782) (5.803491, -46.417148) (5.713834, -46.332868) (5.62589, -46.245784) knots 0 0 0 0 0.90811925 0.90811925 0.90811925 1 1 1 1
  spline S250 degree 3 poles (5.62589, -46.245784) (4.846737, -45.474263) (4.306905, -44.462375) (4.019359, -43.433886) (3.8158, -42.705805) (3.717196, -41.960838) (3.677569, -41.176696) knots 0.00000121 0.00000121 0.00000121 0.00000121 0.58551026 0.58551026 0.58551026 1 1 1 1
  spline S251 degree 3 poles (3.677569, -41.176696) (3.551917, -38.690291) (4.328331, -36.236007) (5.755968, -34.087317) (5.974616, -33.758237) (6.208464, -33.435292) (6.456711, -33.118665) knots 0 0 0 0 0.68431637 0.68431637 0.68431637 0.78912214 0.78912214 0.78912214 0.78912214
  spline S252 degree 3 poles (6.456711, -33.118665) (6.34851, -33.103991) (6.246861, -33.088464) (6.146113, -33.072391) knots 0.85136939 0.85136939 0.85136939 0.85136939 1 1 1 1
  spline S253 degree 3 poles (6.146107, -33.07239) (4.427586, -32.798214) (2.894725, -32.313728) (1.576824, -31.441221) (1.121257, -31.139617) (0.696721, -30.792947) (0.314944, -30.408091) knots 0 0 0 0 0.7431212 0.7431212 0.7431212 1 1 1 1
  spline S254 degree 3 poles (0.314944, -30.408091) (-0.607959, -29.477748) (-1.313273, -28.271903) (-1.642016, -26.983449) (-1.790215, -26.402609) (-1.869991, -25.810839) (-1.898014, -25.215262) knots 0.00000055 0.00000055 0.00000055 0.00000055 0.68927295 0.68927295 0.68927295 1 1 1 1
  spline S255 degree 3 poles (-1.898014, -25.215262) (-1.978761, -23.499116) (-1.620194, -21.790181) (-0.739433, -20.351415) (0.135441, -18.922265) (1.480422, -17.833695) (3.023363, -17.130053) (3.740321, -16.803092) (4.503698, -16.550874) (5.308727, -16.360896) knots 0.00000002 0.00000002 0.00000002 0.00000002 0.4073516 0.4073516 0.4073516 0.81198092 0.81198092 0.81198092 1 1 1 1
  spline S256 degree 3 poles (5.308727, -16.360896) (6.34615, -16.116075) (7.45886, -15.983662) (8.63716, -15.92934) knots 0.00000006 0.00000006 0.00000006 0.00000006 0.34838739 0.34838739 0.34838739 0.34838739
  spline S257 degree 3 poles (8.63716, -15.92934) (7.799543, -14.667397) (7.129059, -13.340524) (6.669682, -11.970846) (6.494849, -11.449561) (6.350924, -10.921934) (6.242066, -10.389024) knots 0.44294636 0.44294636 0.44294636 0.44294636 0.84643618 0.84643618 0.84643618 1 1 1 1
  spline S258 degree 3 poles (6.242066, -10.389024) (5.848143, -8.460593) (5.888073, -6.538054) (6.439741, -4.770172) (6.68202, -3.99376) (7.028243, -3.244145) (7.516165, -2.55628) knots 0.00000002 0.00000002 0.00000002 0.00000002 0.69484173 0.69484173 0.69484173 1 1 1 1
  spline S259 degree 3 poles (7.516165, -2.55628) (8.222961, -1.559851) (9.128556, -0.898855) (10.157525, -0.43672) (10.472899, -0.295078) (10.801911, -0.175209) (11.145898, -0.080977) knots 0 0 0 0 0.76540677 0.76540677 0.76540677 1 1 1 1
  spline S260 degree 3 poles (11.145901, -0.080976) (11.63688, 0.053523) (11.982265, 0.078511) (12.345585, 0.09782) (12.826679, 0.123389) (13.291779, 0.111851) (13.781926, 0.054183) (14.044506, 0.023289) (14.309219, -0.017278) (14.636461, -0.109149) knots 0 0 0 0 0.32964817 0.32964817 0.32964817 0.7661555 0.7661555 0.7661555 1 1 1 1
  spline S261 degree 3 poles (14.636461, -0.109149) (16.201849, -0.548618) (17.515098, -1.481152) (18.696047, -2.668391) (18.853246, -2.826427) (19.00813, -2.989498) (19.161311, -3.157888) knots 0.00000029 0.00000029 0.00000029 0.00000029 0.43083502 0.43083502 0.43083502 0.48818469 0.48818469 0.48818469 0.48818469
  spline S262 degree 3 poles (19.161311, -3.157888) (19.60393, -2.048293) (20.193034, -1.040736) (20.975545, -0.186079) (22.035467, 0.971565) (23.464066, 1.789693) (24.989984, 2.136438) (25.093053, 2.159859) (25.196546, 2.181342) (25.300402, 2.200932) knots 0.20091084 0.20091084 0.20091084 0.20091084 0.52760254 0.52760254 0.52760254 0.9701106 0.9701106 0.9701106 1 1 1 1
  spline S263 degree 3 poles (25.300403, 2.200932) (25.714913, 2.279119) (26.006408, 2.291167) (26.326489, 2.301129) (26.730026, 2.313688) (27.131646, 2.305559) (27.536743, 2.273194) (27.789068, 2.253035) (28.030231, 2.229357) (28.351539, 2.160191) knots 0 0 0 0 0.32829804 0.32829804 0.32829804 0.74219451 0.74219451 0.74219451 1 1 1 1
  spline S264 degree 3 poles (28.351541, 2.160191) (29.709047, 1.867967) (30.996936, 1.132993) (31.922407, 0.093895) (32.798403, -0.889652) (33.358046, -2.087246) (33.690392, -3.370258) knots 0 0 0 0 0.5137321 0.5137321 0.5137321 1 1 1 1
  spline S265 degree 3 poles (33.690392, -3.370258) (33.776473, -3.702566) (33.854687, -4.036898) (33.914278, -4.385894) knots 0.00000103 0.00000103 0.00000103 0.00000103 0.303372 0.303372 0.303372 0.303372
  spline S266 degree 3 poles (33.914278, -4.385894) (35.077591, -3.710105) (36.25615, -3.223399) (37.495135, -3.002336) (37.925506, -2.925548) (38.358461, -2.880919) (38.788292, -2.865561) knots 0.043821 0.043821 0.043821 0.043821 0.753491 0.753491 0.753491 1 1 1 1
  spline S267 degree 3 poles (38.788292, -2.865561) (39.536623, -2.838822) (40.328145, -2.895436) (41.076573, -3.098004) (41.393373, -3.183747) (41.694744, -3.290015) (41.981075, -3.406751) knots 0.00000009 0.00000009 0.00000009 0.00000009 0.70259967 0.70259967 0.70259967 1 1 1 1
  spline S268 degree 3 poles (41.981076, -3.406751) (43.245686, -3.922328) (44.392522, -4.815268) (45.144661, -5.980053) (45.767287, -6.944272) (46.11375, -8.049526) (46.239432, -9.172792) knots 0 0 0 0 0.54710346 0.54710346 0.54710346 1 1 1 1
  spline S269 degree 3 poles (46.239432, -9.172792) (46.377458, -10.406386) (46.194007, -11.546781) (45.871165, -12.682891) (45.532419, -13.874968) (45.019964, -15.041884) (44.303092, -16.108155) knots 0.00000003 0.00000003 0.00000003 0.00000003 0.48798052 0.48798052 0.48798052 1 1 1 1
  spline S270 degree 3 poles (44.303092, -16.108155) (44.164426, -16.314407) (44.019282, -16.517032) (43.867274, -16.718121) knots 0.00000011 0.00000011 0.00000011 0.00000011 0.1564771 0.1564771 0.1564771 0.1564771
  spline S271 degree 3 poles (43.867274, -16.718121) (44.954351, -16.948735) (45.990256, -17.277941) (46.958878, -17.716157) (47.901124, -18.14244) (48.78054, -18.672976) (49.571631, -19.311931) knots 0.47897696 0.47897696 0.47897696 0.47897696 0.74308438 0.74308438 0.74308438 1 1 1 1
  spline S272 degree 3 poles (49.571631, -19.311931) (50.872301, -20.362464) (51.904962, -21.657042) (52.417371, -23.247218) (52.449247, -23.346137) (52.47892, -23.446174) (52.506244, -23.547297) knots 0.00000094 0.00000094 0.00000094 0.00000094 0.94143364 0.94143364 0.94143364 0.99999688 0.99999688 0.99999688 0.99999688
  spline S273 degree 3 poles (52.506244, -23.547297) (52.684533, -24.207119) (52.71534, -24.74605) (52.707508, -25.311253) (52.700708, -25.80199) (52.663485, -26.278502) (52.50775, -26.854446) (52.507744, -26.854467) (52.507738, -26.854488) (52.507733, -26.85451) knots 0 0 0 0 0.53526096 0.53526096 0.53526096 1 1 1 1.00004181 1.00004181 1.00004181 1.00004181
  spline S274 degree 3 poles (52.507733, -26.85451) (52.507727, -26.854531) (52.507721, -26.854553) (52.507715, -26.854574) (52.058989, -28.513755) (51.00835, -29.854923) (49.712862, -30.860796) (48.765997, -31.595983) (47.671156, -32.16563) (46.471596, -32.565691) knots -0.00001316 -0.00001316 -0.00001316 -0.00001316 0 0 0 0.57773623 0.57773623 0.57773623 1 1 1 1
  spline S275 degree 3 poles (46.471596, -32.565691) (45.252937, -32.972123) (43.981019, -33.187663) (42.600211, -33.226398) knots 0.00000022 0.00000022 0.00000022 0.00000022 0.79992155 0.79992155 0.79992155 0.79992155